Autodesk Inventor part; units mm, degrees
(part 3 of 3)
  line L647 (97.7332, -44.3356) -> (111.7794, -30.2894) construction
  line L648 (111.7794, -44.3356) -> (97.7332, -30.2894) construction
  arc A876 (98.038, -30.2894) -> (97.7332, -30.5942) centre (98.038, -30.5942) ccw
  arc A877 (111.7794, -30.5942) -> (111.4746, -30.2894) centre (111.4746, -30.5942) ccw
  arc A878 (111.4746, -44.3356) -> (111.7794, -44.0308) centre (111.4746, -44.0308) ccw
  arc A879 (97.7332, -44.0308) -> (98.038, -44.3356) centre (98.038, -44.0308) ccw
  line L649 (117.088, -44.3356) -> (130.5246, -44.3356)
  line L650 (130.8294, -44.0308) -> (130.8294, -30.5942)
  line L651 (130.5246, -30.2894) -> (117.088, -30.2894)
  line L652 (116.7832, -30.5942) -> (116.7832, -44.0308)
  line L653 (116.7832, -44.3356) -> (130.8294, -30.2894) construction
  line L654 (130.8294, -44.3356) -> (116.7832, -30.2894) construction
  arc A880 (117.088, -30.2894) -> (116.7832, -30.5942) centre (117.088, -30.5942) ccw
  arc A881 (130.8294, -30.5942) -> (130.5246, -30.2894) centre (130.5246, -30.5942) ccw
  arc A882 (130.5246, -44.3356) -> (130.8294, -44.0308) centre (130.5246, -44.0308) ccw
  arc A883 (116.7832, -44.0308) -> (117.088, -44.3356) centre (117.088, -44.0308) ccw
  line L655 (136.1379, -44.3356) -> (149.5746, -44.3356)
  line L656 (149.8794, -44.0308) -> (149.8794, -30.5942)
  line L657 (149.5746, -30.2894) -> (136.1379, -30.2894)
  line L658 (135.8332, -30.5942) -> (135.8332, -44.0308)
  line L659 (135.8332, -44.3356) -> (149.8794, -30.2894) construction
  line L660 (149.8794, -44.3356) -> (135.8332, -30.2894) construction
  arc A884 (136.1379, -30.2894) -> (135.8332, -30.5942) centre (136.1379, -30.5942) ccw
  arc A885 (149.8794, -30.5942) -> (149.5746, -30.2894) centre (149.5746, -30.5942) ccw
  arc A886 (149.5746, -44.3356) -> (149.8794, -44.0308) centre (149.5746, -44.0308) ccw
  arc A887 (135.8332, -44.0308) -> (136.1379, -44.3356) centre (136.138, -44.0308) ccw
  line L661 (112.3255, 12.8144) -> (125.7621, 12.8144)
  line L662 (126.0669, 13.1192) -> (126.0669, 26.5558)
  line L663 (125.7621, 26.8606) -> (112.3255, 26.8606)
  line L664 (112.0207, 26.5558) -> (112.0207, 13.1192)
  line L665 (112.0207, 12.8144) -> (126.0669, 26.8606) construction
  line L666 (126.0669, 12.8144) -> (112.0207, 26.8606) construction
  arc A888 (112.3255, 26.8606) -> (112.0207, 26.5558) centre (112.3255, 26.5558) ccw
  arc A889 (126.0669, 26.5558) -> (125.7621, 26.8606) centre (125.7621, 26.5558) ccw
  arc A890 (125.7621, 12.8144) -> (126.0669, 13.1192) centre (125.7621, 13.1192) ccw
  arc A891 (112.0207, 13.1192) -> (112.3255, 12.8144) centre (112.3255, 13.1192) ccw
  line L667 (90.8942, -25.2856) -> (104.3308, -25.2856)
  line L668 (104.6356, -24.9808) -> (104.6356, -11.5442)
  line L669 (104.3308, -11.2394) -> (90.8942, -11.2394)
  line L670 (90.5894, -11.5442) -> (90.5894, -24.9808)
  line L671 (90.5894, -25.2856) -> (104.6356, -11.2394) construction
  line L672 (104.6356, -25.2856) -> (90.5894, -11.2394) construction
  arc A892 (90.8942, -11.2394) -> (90.5894, -11.5442) centre (90.8942, -11.5442) ccw
  arc A893 (104.6356, -11.5442) -> (104.3308, -11.2394) centre (104.3308, -11.5442) ccw
  arc A894 (104.3308, -25.2856) -> (104.6356, -24.9808) centre (104.3308, -24.9808) ccw
  arc A895 (90.5894, -24.9808) -> (90.8942, -25.2856) centre (90.8942, -24.9808) ccw
  line L673 (107.5757, 45.8979) -> (120.9869, 45.8979)
  line L674 (121.2917, 45.5931) -> (121.2917, 32.1819)
  line L675 (120.9869, 31.8771) -> (107.5757, 31.8771)
  line L676 (107.2709, 32.1819) -> (107.2709, 45.5931)
  line L677 (107.2709, 45.8979) -> (121.2917, 31.8771) construction
  line L678 (121.2917, 45.8979) -> (107.2709, 31.8771) construction
  line L679 (114.2813, 45.8979) -> (114.2813, 31.8771)
  arc A896 (107.5757, 45.8979) -> (107.2709, 45.5931) centre (107.5757, 45.5931) ccw
  arc A897 (121.2917, 45.5931) -> (120.9869, 45.8979) centre (120.9869, 45.5931) ccw
  arc A898 (120.9869, 31.8771) -> (121.2917, 32.1819) centre (120.9869, 32.1819) ccw
  arc A899 (107.2709, 32.1819) -> (107.5757, 31.8771) centre (107.5757, 32.1819) ccw
  line L680 (114.2813, 38.8875) -> (102.2925, 38.8875)
  line L681 (105.6707, 45.0851) -> (105.6706, 44.1707)
  line L682 (98.9143, 45.0851) -> (105.6707, 45.0851)
  line L683 (100.7177, 31.4707) -> (103.8673, 31.4707)
  line L684 (103.8673, 31.4707) -> (103.8673, 32.6899)
  line L685 (103.8673, 32.6899) -> (105.6707, 32.6899)
  line L686 (105.6707, 32.6899) -> (105.6706, 33.5789)
  line L687 (100.7177, 32.6899) -> (100.7177, 31.4707)
  line L688 (98.9143, 45.0851) -> (98.9143, 41.8847)
  line L689 (98.9143, 41.8847) -> (97.9745, 41.8847)
  line L690 (97.9745, 38.8875) -> (98.9143, 38.8875)
  line L691 (97.9745, 41.8847) -> (97.9745, 38.8875)
  line L692 (105.6706, 33.5789) -> (105.6706, 44.1707)
  line L693 (98.9143, 45.0851) -> (105.6707, 32.6899) construction
  line L694 (105.6707, 45.0851) -> (98.9143, 32.6899) construction
  line L695 (102.2925, 45.0851) -> (102.2925, 31.4707)
  line L696 (98.9143, 38.8875) -> (98.9143, 32.6899)
  line L697 (98.9143, 32.6899) -> (100.7177, 32.6899)
  line L698 (105.6706, 33.5789) -> (107.2709, 33.5789)
  line L699 (105.6706, 44.1707) -> (107.2709, 44.1707)
  line L700 (129.6483, 38.8875) -> (129.6483, 32.6899)
  line L701 (130.5881, 38.8875) -> (129.6483, 38.8875)
  line L702 (126.27, 45.0851) -> (126.27, 31.4707)
  line L703 (122.8919, 33.5789) -> (122.8919, 44.1707)
  line L704 (129.6483, 45.0851) -> (122.8919, 32.6899) construction
  line L705 (122.8919, 45.0851) -> (129.6483, 32.6899) construction
  line L706 (130.5881, 41.8847) -> (130.5881, 38.8875)
  line L707 (129.6483, 32.6899) -> (127.8449, 32.6899)
  line L708 (127.8449, 32.6899) -> (127.8449, 31.4707)
  line L709 (122.8919, 32.6899) -> (122.8919, 33.5789)
  line L710 (124.6953, 31.4707) -> (124.6953, 32.6899)
  line L711 (127.8449, 31.4707) -> (124.6953, 31.4707)
  line L712 (124.6953, 32.6899) -> (122.8919, 32.6899)
  line L713 (129.6483, 41.8847) -> (130.5881, 41.8847)
  line L714 (129.6483, 45.0851) -> (129.6483, 41.8847)
  line L715 (129.6483, 45.0851) -> (122.8919, 45.0851)
  line L716 (122.8919, 45.0851) -> (122.8919, 44.1707)
  line L717 (114.2813, 38.8875) -> (126.27, 38.8875)
  line L718 (-137.6931, -11.2521) -> (-124.2819, -11.2521)
  line L719 (-123.9771, -11.5569) -> (-123.9771, -24.9681)
  line L720 (-124.2819, -25.2729) -> (-137.6931, -25.2729)
  line L721 (-137.9979, -24.9681) -> (-137.9979, -11.5569)
  line L722 (-137.9979, -11.2521) -> (-123.9771, -25.2729) construction
  line L723 (-123.9771, -11.2521) -> (-137.9979, -25.2729) construction
  line L724 (-130.9875, -11.2521) -> (-130.9875, -25.2729)
  arc A900 (-137.6931, -11.2521) -> (-137.9979, -11.5569) centre (-137.6931, -11.5569) ccw
  arc A901 (-123.9771, -11.5569) -> (-124.2819, -11.2521) centre (-124.2819, -11.5569) ccw
  arc A902 (-124.2819, -25.2729) -> (-123.9771, -24.9681) centre (-124.2819, -24.9681) ccw
  arc A903 (-137.9979, -24.9681) -> (-137.6931, -25.2729) centre (-137.6931, -24.9681) ccw
  line L725 (-130.9875, -18.2625) -> (-142.9763, -18.2625)
  line L726 (-139.5981, -12.0649) -> (-139.5981, -12.9793)
  line L727 (-146.3545, -12.0649) -> (-139.5981, -12.0649)
  line L728 (-144.5511, -25.6793) -> (-141.4015, -25.6793)
  line L729 (-141.4015, -25.6793) -> (-141.4015, -24.4601)
  line L730 (-141.4015, -24.4601) -> (-139.5981, -24.4601)
  line L731 (-139.5981, -24.4601) -> (-139.5981, -23.5711)
  line L732 (-144.5511, -24.4601) -> (-144.5511, -25.6793)
  line L733 (-146.3545, -12.0649) -> (-146.3545, -15.2653)
  line L734 (-146.3545, -15.2653) -> (-147.2943, -15.2653)
  line L735 (-147.2943, -18.2625) -> (-146.3545, -18.2625)
  line L736 (-147.2943, -15.2653) -> (-147.2943, -18.2625)
  line L737 (-139.5981, -23.5711) -> (-139.5981, -12.9793)
  line L738 (-146.3545, -12.0649) -> (-139.5981, -24.4601) construction
  line L739 (-139.5981, -12.0649) -> (-146.3545, -24.4601) construction
  line L740 (-142.9763, -12.0649) -> (-142.9763, -25.6793)
  line L741 (-146.3545, -18.2625) -> (-146.3545, -24.4601)
  line L742 (-146.3545, -24.4601) -> (-144.5511, -24.4601)
  line L743 (-139.5981, -23.5711) -> (-137.9979, -23.5711)
  line L744 (-139.5981, -12.9793) -> (-137.9979, -12.9793)
  line L745 (-115.6205, -18.2625) -> (-115.6205, -24.4601)
  line L746 (-114.6807, -18.2625) -> (-115.6205, -18.2625)
  line L747 (-118.9987, -12.0649) -> (-118.9987, -25.6793)
  line L748 (-122.3769, -23.5711) -> (-122.3769, -12.9793)
  line L749 (-115.6205, -12.0649) -> (-122.3769, -24.4601) construction
  line L750 (-122.3769, -12.0649) -> (-115.6205, -24.4601) construction
  line L751 (-114.6807, -15.2653) -> (-114.6807, -18.2625)
  line L752 (-115.6205, -24.4601) -> (-117.4239, -24.4601)
  line L753 (-117.4239, -24.4601) -> (-117.4239, -25.6793)
  line L754 (-122.3769, -24.4601) -> (-122.3769, -23.5711)
  line L755 (-120.5735, -25.6793) -> (-120.5735, -24.4601)
  line L756 (-117.4239, -25.6793) -> (-120.5735, -25.6793)
  line L757 (-120.5735, -24.4601) -> (-122.3769, -24.4601)
  line L758 (-115.6205, -15.2653) -> (-114.6807, -15.2653)
  line L759 (-115.6205, -12.0649) -> (-115.6205, -15.2653)
  line L760 (-115.6205, -12.0649) -> (-122.3769, -12.0649)
  line L761 (-122.3769, -12.0649) -> (-122.3769, -12.9793)
  line L762 (-130.9875, -18.2625) -> (-118.9987, -18.2625)
  line L763 (105.1944, 7.7979) -> (118.6056, 7.7979)
  line L764 (118.9104, 7.4931) -> (118.9104, -5.9181)
  line L765 (118.6056, -6.2229) -> (105.1944, -6.2229)
  line L766 (104.8896, -5.9181) -> (104.8896, 7.4931)
  line L767 (104.8896, 7.7979) -> (118.9104, -6.2229) construction
  line L768 (118.9104, 7.7979) -> (104.8896, -6.2229) construction
  line L769 (111.9, 7.7979) -> (111.9, -6.2229)
  arc A904 (105.1944, 7.7979) -> (104.8896, 7.4931) centre (105.1944, 7.4931) ccw
  arc A905 (118.9104, 7.4931) -> (118.6056, 7.7979) centre (118.6056, 7.4931) ccw
  arc A906 (118.6056, -6.2229) -> (118.9104, -5.9181) centre (118.6056, -5.9181) ccw
  arc A907 (104.8896, -5.9181) -> (105.1944, -6.2229) centre (105.1944, -5.9181) ccw
  line L770 (111.9, 0.7875) -> (99.9112, 0.7875)
  line L771 (103.2894, 6.9851) -> (103.2894, 6.0707)
  line L772 (96.533, 6.9851) -> (103.2894, 6.9851)
  line L773 (98.3364, -6.6293) -> (101.486, -6.6293)
  line L774 (101.486, -6.6293) -> (101.486, -5.4101)
  line L775 (101.486, -5.4101) -> (103.2894, -5.4101)
  line L776 (103.2894, -5.4101) -> (103.2894, -4.5211)
  line L777 (98.3364, -5.4101) -> (98.3364, -6.6293)
  line L778 (96.533, 6.9851) -> (96.533, 3.7847)
  line L779 (96.533, 3.7847) -> (95.5932, 3.7847)
  line L780 (95.5932, 0.7875) -> (96.533, 0.7875)
  line L781 (95.5932, 3.7847) -> (95.5932, 0.7875)
  line L782 (103.2894, -4.5211) -> (103.2894, 6.0707)
  line L783 (96.533, 6.9851) -> (103.2894, -5.4101) construction
  line L784 (103.2894, 6.9851) -> (96.533, -5.4101) construction
  line L785 (99.9112, 6.9851) -> (99.9112, -6.6293)
  line L786 (96.533, 0.7875) -> (96.533, -5.4101)
  line L787 (96.533, -5.4101) -> (98.3364, -5.4101)
  line L788 (103.2894, -4.5211) -> (104.8896, -4.5211)
  line L789 (103.2894, 6.0707) -> (104.8896, 6.0707)
  line L790 (127.267, 0.7875) -> (127.267, -5.4101)
  line L791 (128.2068, 0.7875) -> (127.267, 0.7875)
  line L792 (123.8888, 6.9851) -> (123.8888, -6.6293)
  line L793 (120.5106, -4.5211) -> (120.5106, 6.0707)
  line L794 (127.267, 6.9851) -> (120.5106, -5.4101) construction
  line L795 (120.5106, 6.9851) -> (127.267, -5.4101) construction
  line L796 (128.2068, 3.7847) -> (128.2068, 0.7875)
  line L797 (127.267, -5.4101) -> (125.4636, -5.4101)
  line L798 (125.4636, -5.4101) -> (125.4636, -6.6293)
  line L799 (120.5106, -5.4101) -> (120.5106, -4.5211)
  line L800 (122.314, -6.6293) -> (122.314, -5.4101)
  line L801 (125.4636, -6.6293) -> (122.314, -6.6293)
  line L802 (122.314, -5.4101) -> (120.5106, -5.4101)
  line L803 (127.267, 3.7847) -> (128.2068, 3.7847)
  line L804 (127.267, 6.9851) -> (127.267, 3.7847)
  line L805 (127.267, 6.9851) -> (120.5106, 6.9851)
  line L806 (120.5106, 6.9851) -> (120.5106, 6.0707)
  line L807 (111.9, 0.7875) -> (123.8888, 0.7875)
  line L808 (-28.1556, -44.3229) -> (-14.7444, -44.3229)
  line L809 (-14.4396, -44.0181) -> (-14.4396, -30.6069)
  line L810 (-14.7444, -30.3021) -> (-28.1556, -30.3021)
  line L811 (-28.4604, -30.6069) -> (-28.4604, -44.0181)
  line L812 (-28.4604, -44.3229) -> (-14.4396, -30.3021) construction
  line L813 (-14.4396, -44.3229) -> (-28.4604, -30.3021) construction
  arc A908 (-28.1556, -30.3021) -> (-28.4604, -30.6069) centre (-28.1556, -30.6069) ccw
  arc A909 (-14.4396, -30.6069) -> (-14.7444, -30.3021) centre (-14.7444, -30.6069) ccw
  arc A910 (-14.7444, -44.3229) -> (-14.4396, -44.0181) centre (-14.7444, -44.0181) ccw
  arc A911 (-28.4604, -44.0181) -> (-28.1556, -44.3229) centre (-28.1556, -44.0181) ccw
  line L814 (-21.45, -37.3125) -> (-71.4499, -37.3125)
  line L815 (-74.8281, -34.3153) -> (-75.7679, -34.3153)
  line L816 (-68.0717, -31.1149) -> (-68.0717, -32.0293)
  line L817 (-74.8281, -31.1149) -> (-68.0717, -31.1149)
  line L818 (-74.8281, -31.1149) -> (-74.8281, -34.3153)
  line L819 (-68.0717, -43.5101) -> (-68.0717, -42.6211)
  line L820 (-68.0717, -42.6211) -> (-68.0717, -32.0293)
  line L821 (-75.7679, -37.3125) -> (-74.8281, -37.3125)
  line L822 (-75.7679, -34.3153) -> (-75.7679, -37.3125)
  line L823 (-68.0717, -31.1149) -> (-74.8281, -43.5101) construction
  line L824 (-74.8281, -31.1149) -> (-68.0717, -43.5101) construction
  line L825 (-71.4499, -31.1149) -> (-71.4499, -44.7293)
  line L826 (-74.8281, -37.3125) -> (-74.8281, -43.5101)
  line L827 (-74.8281, -43.5101) -> (-73.0247, -43.5101)
  line L828 (-69.8751, -43.5101) -> (-68.0717, -43.5101)
  line L829 (-73.0247, -43.5101) -> (-73.0247, -44.7293)
  line L830 (-73.0247, -44.7293) -> (-69.8751, -44.7293)
  line L831 (-69.8751, -44.7293) -> (-69.8751, -43.5101)
  line L832 (-64.8239, -37.3125) -> (-64.8239, -35.0625)
  line L833 (-62.8681, -37.3125) -> (-62.8681, -39.5625)
  line L834 (-21.45, -30.3021) -> (-21.45, -44.3229)
  line L835 (-68.0717, -35.0625) -> (-21.45, -35.0625)
  line L836 (-68.0717, -39.5625) -> (-21.45, -39.5625)
  line L837 (25.1717, -31.1149) -> (25.1717, -32.0293)
  line L838 (25.1717, -42.6211) -> (25.1717, -32.0293)
  line L839 (25.1717, -43.5101) -> (25.1717, -42.6211)
  line L840 (32.8679, -34.3153) -> (32.8679, -37.3125)
  line L841 (32.8679, -37.3125) -> (31.9281, -37.3125)
  line L842 (31.9281, -37.3125) -> (31.9281, -43.5101)
  line L843 (31.9281, -34.3153) -> (32.8679, -34.3153)
  line L844 (31.9281, -31.1149) -> (31.9281, -34.3153)
  line L845 (31.9281, -43.5101) -> (30.1247, -43.5101)
  line L846 (30.1247, -43.5101) -> (30.1247, -44.7293)
  line L847 (28.5499, -31.1149) -> (28.5499, -44.7293)
  line L848 (30.1247, -44.7293) -> (26.9751, -44.7293)
  line L849 (26.9751, -44.7293) -> (26.9751, -43.5101)
  line L850 (26.9751, -43.5101) -> (25.1717, -43.5101)
  line L851 (25.1717, -31.1149) -> (31.9281, -43.5101) construction
  line L852 (31.9281, -31.1149) -> (25.1717, -43.5101) construction
  line L853 (31.9281, -31.1149) -> (25.1717, -31.1149)
  line L854 (25.1717, -35.0625) -> (-21.45, -35.0625)
  line L855 (-21.45, -37.3125) -> (28.5499, -37.3125)
  line L856 (25.1717, -39.5625) -> (-21.45, -39.5625)
  line L857 (-159.6, -70.7) -> (159.6, -70.7)
  line L858 (159.6, -70.7) -> (159.6, -83.4)
  line L859 (159.6, -83.4) -> (-159.6, -83.4)
  line L860 (-159.6, -83.4) -> (-159.6, -70.7)
  line L861 (-159.6, -83.4) -> (159.6, -83.4)
  line L862 (159.6, -83.4) -> (159.6, -96.1)
  line L863 (159.6, -96.1) -> (-159.6, -96.1)
  line L864 (-159.6, -96.1) -> (-159.6, -83.4)
  line L865 (-159.6, 70.7) -> (159.6, 70.7)
  line L866 (159.6, 70.7) -> (159.6, 93.56)
  line L867 (159.6, 93.56) -> (-159.6, 93.56)
  line L868 (-159.6, 93.56) -> (-159.6, 70.7)
  line L869 (-159.6, 93.56) -> (159.6, 93.56)
  line L870 (159.6, 93.56) -> (159.6, 106.26)
  line L871 (159.6, 106.26) -> (-159.6, 106.26)
  line L872 (-159.6, 106.26) -> (-159.6, 93.56)
  line L873 (-137.2245, 70.7) -> (-137.2245, 73.24)
  line L874 (-129.196, 70.7) -> (-129.196, 73.24)
  line L875 (-137.2245, 73.24) -> (-129.196, 73.24)
  line L876 (-129.196, 73.24) -> (-129.196, 79.59)
  line L877 (-129.196, 79.59) -> (-137.2245, 79.59)
  line L878 (-137.2245, 79.59) -> (-137.2245, 73.24)
  line L879 (107.2709, 44.1707) -> (122.8919, 44.1707)
  line L880 (107.2709, 33.5789) -> (122.8919, 33.5789)
  line L881 (104.8896, 6.0707) -> (120.5106, 6.0707)
  line L882 (104.8896, -4.5211) -> (120.5106, -4.5211)
  line L883 (-137.9979, -12.9793) -> (-122.3769, -12.9793)
  line L884 (-137.9979, -23.5711) -> (-122.3769, -23.5711)
  point P0 (0, 0)
  point P1 (-47.6438, 38.8875)
  point P2 (-9.5437, 38.8875)
  point P3 (-47.6438, 38.8875)
  point P4 (-9.5437, 38.8875)
  point P5 (-76.2188, 19.8375)
  point P6 (-57.1688, 19.8375)
  point P7 (-38.1188, 19.8375)
  point P8 (-0.0188, 19.8375)
  point P9 (-109.5563, 0.7875)
  point P10 (-90.5062, 0.7875)
  point P11 (-71.4563, 0.7875)
  point P12 (-52.4062, 0.7875)
  point P13 (-33.3563, 0.7875)
  point P14 (-14.3063, 0.7875)
  point P15 (4.7438, 0.7875)
  point P16 (23.7937, 0.7875)
  point P17 (42.8438, 0.7875)
  point P18 (61.8937, 0.7875)
  point P19 (80.9437, 0.7875)
  point P20 (142.8562, 0.7875)
  point P21 (-61.989, -18.2047)
  point P22 (-23.8312, -18.2625)
  point P23 (-4.7813, -18.2625)
  point P24 (14.2687, -18.2625)
  point P25 (-140.5125, -37.3125)
  point P26 (-116.7, -37.3125)
  point P27 (-92.8875, -37.3125)
  point P28 (47.6063, -37.3125)
  point P29 (-138.1313, 19.8375)
  point P30 (-135.75, 0.7875)
  point P31 (66.6562, -37.3125)
  point P32 (85.7062, -37.3125)
  point P33 (104.7563, -37.3125)
  point P34 (123.8063, -37.3125)
  point P35 (142.8562, -37.3125)
  point P36 (-71.4499, -37.3125)
  point P37 (28.5499, -37.3125)
  point P38 (156.425, -45.7916)
  point P39 (-156.425, 48.1608)
  dimension "d0" = 301
  dimension "d1" = 108.5
  dimension "d2" = 12.7
  dimension "d3" = 6.35
  dimension "d4" = 6.35
  dimension "d5" = 12.7
  dimension "d6" = 141.4
  dimension "d31" = 14.0462
  dimension "d32" = 14.0462
  dimension "d33" = 0.3048
  dimension "d34" = 0.3048
  dimension "d35" = 0.3048
  dimension "d36" = 0.3048
  dimension "d37" = 14.0462
  dimension "d38" = 14.0462
  dimension "d39" = 0.3048
  dimension "d40" = 0.3048
  dimension "d41" = 0.3048
  dimension "d42" = 0.3048
  dimension "d43" = 14.0462
  dimension "d44" = 14.0462
  dimension "d45" = 0.3048
  dimension "d46" = 0.3048
  dimension "d47" = 0.3048
  dimension "d48" = 0.3048
  dimension "d49" = 14.0462
  dimension "d50" = 14.0462
  dimension "d51" = 0.3048
  dimension "d52" = 0.3048
  dimension "d53" = 0.3048
  dimension "d54" = 0.3048
  dimension "d55" = 14.0462
  dimension "d56" = 14.0462
  dimension "d57" = 0.3048
  dimension "d58" = 0.3048
  dimension "d59" = 0.3048
  dimension "d60" = 0.3048
  dimension "d61" = 14.0462
  dimension "d62" = 14.0462
  dimension "d63" = 0.3048
  dimension "d64" = 0.3048
  dimension "d65" = 0.3048
  dimension "d66" = 0.3048
  dimension "d67" = 14.0462
  dimension "d68" = 14.0462
  dimension "d69" = 0.3048
  dimension "d70" = 0.3048
  dimension "d71" = 0.3048
  dimension "d72" = 0.3048
  dimension "d73" = 14.0462
  dimension "d74" = 14.0462
  dimension "d75" = 0.3048
  dimension "d76" = 0.3048
  dimension "d77" = 0.3048
  dimension "d78" = 0.3048
  dimension "d79" = 14.0462
  dimension "d80" = 14.0462
  dimension "d81" = 0.3048
  dimension "d82" = 0.3048
  dimension "d83" = 0.3048
  dimension "d84" = 0.3048
  dimension "d85" = 14.0462
  dimension "d86" = 14.0462
  dimension "d87" = 0.3048
  constraints: 1770 end point, 1104 point on circle, 912 centre point, 564 point on line, 544 tangent, 167 midpoint, 149 parallel, 93 horizontal, 92 perpendicular, 74 symmetric about line, 25 vertical, 12 collinear, 3 other
  measures "d0" distance of L4.start L4.end
  measures "d1" distance of L2.end L3.end
  measures "d2" distance of L281.start L281.end
  measures "d3" distance of L282.start L282.end
  measures "d4" distance of L284.start L284.end
  measures "d5" distance of L283.start L283.end
  measures "d6" distance of L285.end L286.end
  measures "d31" distance of L293.end L294.end
  measures "d32" distance of L294.start L293.end
  measures "d33" radius of A640
  measures "d34" radius of A641
  measures "d35" radius of A642
  measures "d36" radius of A643
  measures "d37" distance of L299.end L300.end
  measures "d38" distance of L300.start L299.end
  measures "d39" radius of A644
  measures "d40" radius of A645
  measures "d41" radius of A646
  measures "d42" radius of A647
  measures "d43" distance of L305.end L306.end
  measures "d44" distance of L306.start L305.end
  measures "d45" radius of A648
  measures "d46" radius of A649
  measures "d47" radius of A650
  measures "d48" radius of A651
  measures "d49" distance of L311.end L312.end
  measures "d50" distance of L312.start L311.end
  measures "d51" radius of A652
  measures "d52" radius of A653
  measures "d53" radius of A654
  measures "d54" radius of A655
  measures "d55" distance of L317.end L318.end
  measures "d56" distance of L318.start L317.end
  measures "d57" radius of A656
  measures "d58" radius of A657
  measures "d59" radius of A658
  measures "d60" radius of A659
  measures "d61" distance of L323.end L324.end
  measures "d62" distance of L324.start L323.end
  measures "d63" radius of A660
  measures "d64" radius of A661
  measures "d65" radius of A662
  measures "d66" radius of A663
  measures "d67" distance of L329.end L330.end
  measures "d68" distance of L330.start L329.end
  measures "d69" radius of A664
  measures "d70" radius of A665
  measures "d71" radius of A666
  measures "d72" radius of A667
  measures "d73" distance of L335.end L336.end
  measures "d74" distance of L336.start L335.end
  measures "d75" radius of A668
  measures "d76" radius of A669
  measures "d77" radius of A670
  measures "d78" radius of A671
  measures "d79" distance of L341.end L342.end
  measures "d80" distance of L342.start L341.end
  measures "d81" radius of A672
  measures "d82" radius of A673
  measures "d83" radius of A674
  measures "d84" radius of A675
  measures "d85" distance of L347.end L348.end
  measures "d86" distance of L348.start L347.end
  measures "d87" radius of A676
extrude "Plate1" add sketch "Sketch1" along normal blind 3.048 contours A3 L4 A2 L3 L2 A1 L1 A0 L0 | L0 L282 L288 L285 L281 L4 A3 | L0 A0 L1 L283 L287 L288 L282 | L281 L285 L286 L284 L3 A2 L4 | L287 L858 L859 L860 | L868 L867 L866 L285 L874 L876 L877 L878 L873 | L1 A1 L2 L3 L284 L286 L287 L283 | L859 L862 L863 L864 | L872 L871 L870 L867 | L873 L875 L874 L285 | L9 A8 L10 A9 | L11 A10 L12 A11
fold "Fold1" angle 90 bend radius 3.048 thickness 3.048 k factor 0.44 line from (159.6, 0, -83.4) to (-159.6, 0, -83.4) line at bend end moving side (0, 0, -1) folds toward (0, -1, 0)
fold "Fold2" angle 84.678 bend radius 3.048 thickness 3.048 k factor 0.44 line from (-159.6, 0, -70.7) to (159.6, 0, -70.7) line at bend centre moving side (0, 0, -1) folds toward (0, -1, 0)
fold "Fold3" angle 90 bend radius 3.048 thickness 3.048 k factor 0.44 line from (159.6, 0, 93.56) to (-159.6, 0, 93.56) line at bend centre moving side (0, 0, 1) folds toward (0, -1, 0)
fold "Fold4" angle 95.303 bend radius 3.048 thickness 3.048 k factor 0.44 line from (159.6, 0, 70.7) to (-159.6, 0, 70.7) line at bend centre moving side (0, 0, 1) folds toward (0, -1, 0)
hole "Hole1" at (140.5, 3.048, -52.5) direction (0, -1, 0) diameter 4.3 depth 3.048 tip angle 118 countersink diameter 7.5 countersink angle 90
hole "Hole2" at (144.75, 3.048, 52.5) direction (0, -1, 0) diameter 4.3 depth 3.048 tip angle 118 countersink diameter 7.5 countersink angle 90
hole "Hole3" at (-143, 3.048, 52.5) direction (0, -1, 0) diameter 4.3 depth 3.048 tip angle 118 countersink diameter 7.5 countersink angle 90
hole "Hole4" at (-143, 3.048, -52) direction (0, -1, 0) diameter 4.3 depth 3.048 tip angle 118 countersink diameter 7.5 countersink angle 90
body "Solid2"
